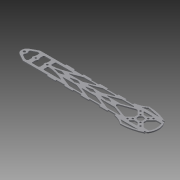
# Autodesk Inventor part: Arm
Saved by Autodesk Inventor 2014 SP1 (Build 180222100, 222)
## iProperties
Created: 2014-07-26
Part Number: Arm
Material: Generic
Document SubType Name: Modeling
Designer: Ryan
Density: 1 g/cm^3
Appearance: Default
Author: Ryan
Autodesk Inventor part; units mm, degrees
ref_plane "YZ Plane" through (0, 0, 0) normal (1, 0, 0) x (0, 1, 0)
ref_plane "XZ Plane" through (0, 0, 0) normal (0, 1, 0) x (-1, 0, 0)
ref_plane "XY Plane" through (0, 0, 0) normal (0, 0, 1) x (1, 0, 0)
sketch "DWG" plane through (0, 0, 0) normal (0, 0, 1) x (1, 0, 0)
  arc A0 (4.5611, 40.079) -> (0, 25.5088) centre (25.5524, 25.5088) ccw construction
  arc A1 (5.3826, 40.5088) -> (4.5611, 40.079) centre (5.3826, 39.5088) ccw construction
  line L0 (5.3826, 40.5088) -> (8.9844, 40.5088) construction
  line L1 (8.9844, 42.5088) -> (5.9833, 42.5088) construction
  arc A2 (41.2735, 51.0175) -> (5.9833, 42.5088) centre (43.8792, -37.2276) ccw construction
  arc A3 (41.2735, 51.0175) -> (59.244, 43.0088) centre (65.3633, 80.9055) ccw construction
  line L2 (222.3706, 39.9043) -> (233.741, 33.7395) construction
  line L3 (177.3927, 40.5088) -> (219.9874, 40.5088) construction
  arc A4 (222.3706, 39.9043) -> (219.9874, 40.5088) centre (219.9874, 35.5088) ccw construction
  arc A5 (0, 25.5088) -> (4.5611, 10.9385) centre (25.5524, 25.5088) ccw construction
  arc A6 (4.5611, 10.9385) -> (5.3826, 10.5088) centre (5.3826, 11.5088) ccw construction
  line L4 (5.3826, 10.5088) -> (8.9839, 10.5088) construction
  line L5 (8.9838, 8.5088) -> (5.9875, 8.5088) construction
  arc A7 (5.9875, 8.5088) -> (41.2735, 0) centre (43.8737, 88.2038) ccw construction
  arc A8 (59.244, 8.0088) -> (41.2735, 0) centre (65.3633, -29.888) ccw construction
  line L6 (222.3706, 11.1132) -> (233.741, 17.278) construction
  line L7 (177.3921, 10.5093) -> (219.9874, 10.5088) construction
  arc A9 (219.9874, 10.5088) -> (222.3706, 11.1132) centre (219.9874, 15.5088) ccw construction
  circle A10 centre (37.7725, 32.248) radius 1.6 construction
  circle A11 centre (24.3375, 18.813) radius 1.6 construction
  circle A12 centre (25.3982, 31.1874) radius 1.6 construction
  circle A13 centre (36.7119, 19.8736) radius 1.6 construction
  circle A14 centre (31.055, 25.5117) radius 5 construction
  line L8 (6.7874, 36.5088) -> (12.7618, 36.5088) construction
  arc A15 (16.2903, 35.0513) -> (12.7618, 36.5088) centre (12.7618, 31.5088) ccw construction
  line L9 (6.7874, 14.5088) -> (12.7425, 14.5088) construction
  arc A16 (12.7425, 14.5088) -> (16.278, 15.9732) centre (12.7425, 19.5088) ccw construction
  circle A17 centre (233.741, 25.5088) radius 2.1 construction
  circle A18 centre (193.7046, 25.5088) radius 1.6 construction
  circle A19 centre (213.981, 25.5088) radius 1.6 construction
  line L10 (199.0246, 36.3758) -> (208.661, 36.3758) construction
  arc A20 (199.0246, 36.3758) -> (197.1246, 34.4758) centre (199.0246, 34.4758) ccw construction
  line L11 (197.1246, 34.4758) -> (197.1246, 28.9288) construction
  line L12 (210.561, 28.9288) -> (210.561, 34.4758) construction
  arc A21 (210.561, 34.4758) -> (208.661, 36.3758) centre (208.661, 34.4758) ccw construction
  line L13 (199.0246, 14.6417) -> (208.661, 14.6417) construction
  arc A22 (197.1246, 16.5417) -> (199.0246, 14.6417) centre (199.0246, 16.5417) ccw construction
  line L14 (197.1246, 16.5417) -> (197.1246, 22.0888) construction
  line L15 (210.561, 22.0888) -> (210.561, 16.5417) construction
  arc A23 (208.661, 14.6417) -> (210.561, 16.5417) centre (208.661, 16.5417) ccw construction
  arc A24 (197.1246, 22.0888) -> (197.1246, 28.9288) centre (193.6586, 25.5088) ccw construction
  arc A25 (210.561, 28.9288) -> (210.561, 22.0888) centre (213.981, 25.5088) ccw construction
  line L16 (221.1675, 36.3758) -> (219.301, 36.3758) construction
  line L17 (217.401, 28.9288) -> (217.401, 34.4758) construction
  arc A26 (219.301, 36.3758) -> (217.401, 34.4758) centre (219.301, 34.4758) ccw construction
  arc A27 (217.401, 22.0888) -> (217.401, 28.9288) centre (213.981, 25.5088) ccw construction
  line L18 (222.0731, 36.1461) -> (229.3266, 32.2135) construction
  arc A28 (222.0731, 36.1461) -> (221.1675, 36.3758) centre (221.1675, 34.4758) ccw construction
  line L19 (230.321, 30.5432) -> (230.321, 28.9288) construction
  arc A29 (230.321, 30.5432) -> (229.3266, 32.2135) centre (228.421, 30.5432) ccw construction
  arc A30 (230.321, 28.9288) -> (230.321, 22.0888) centre (233.741, 25.5088) ccw construction
  line L20 (221.1675, 14.6417) -> (219.301, 14.6417) construction
  line L21 (217.401, 22.0888) -> (217.401, 16.5417) construction
  arc A31 (217.401, 16.5417) -> (219.301, 14.6417) centre (219.301, 16.5417) ccw construction
  line L22 (222.0731, 14.8714) -> (229.3266, 18.804) construction
  arc A32 (221.1675, 14.6417) -> (222.0731, 14.8714) centre (221.1675, 16.5417) ccw construction
  line L23 (230.321, 20.4743) -> (230.321, 22.0888) construction
  arc A33 (229.3266, 18.804) -> (230.321, 20.4743) centre (228.421, 20.4743) ccw construction
  arc A34 (233.741, 17.278) -> (233.741, 33.7395) centre (229.1559, 25.5088) ccw construction
  line L24 (16.9699, 44.0088) -> (46.9493, 44.0088) construction
  arc A35 (40.3396, 48.7188) -> (16.9395, 44.204) centre (47.756, -52.6194) ccw construction
  arc A36 (16.9395, 44.204) -> (16.9699, 44.0088) centre (16.9699, 44.1088) ccw construction
  arc A37 (40.4838, 48.6716) -> (46.9971, 44.1966) centre (65.3633, 77.9055) ccw construction
  arc A38 (40.4838, 48.6716) -> (40.3396, 48.7188) centre (40.3542, 48.5193) ccw construction
  arc A39 (46.9493, 44.0088) -> (46.9971, 44.1966) centre (46.9493, 44.1088) ccw construction
  line L25 (16.9699, 7.0088) -> (46.9493, 7.0088) construction
  arc A40 (16.9395, 6.8135) -> (40.3396, 2.2987) centre (47.756, 103.637) ccw construction
  arc A41 (16.9699, 7.0088) -> (16.9395, 6.8135) centre (16.9699, 6.9088) ccw construction
  arc A42 (40.3396, 2.2987) -> (40.4838, 2.3459) centre (40.3542, 2.4982) ccw construction
  arc A43 (46.9971, 6.8209) -> (40.4838, 2.3459) centre (65.3633, -26.888) ccw construction
  arc A44 (46.9971, 6.8209) -> (46.9493, 7.0088) centre (46.9493, 6.9088) ccw construction
  circle A45 centre (19.7413, 36.8442) radius 1.6 construction
  circle A46 centre (42.3687, 36.8442) radius 1.6 construction
  circle A47 centre (19.7413, 14.2168) radius 1.6 construction
  circle A48 centre (42.3687, 14.2168) radius 1.6 construction
  arc A49 (88.4057, 36.5567) -> (104.0793, 30.6226) centre (168.1638, 223.554) ccw construction
  arc A50 (104.0793, 30.6226) -> (104.7095, 30.5207) centre (104.7098, 32.5207) ccw construction
  arc A51 (88.7983, 38.4766) -> (88.4057, 36.5567) centre (88.798, 37.4766) ccw construction
  arc A52 (109.7552, 38.3866) -> (127.7097, 31.4923) centre (191.5259, 224.5125) ccw construction
  arc A53 (127.5526, 30.5176) -> (127.7097, 31.4923) centre (127.5527, 31.0176) ccw construction
  arc A54 (109.7552, 38.3866) -> (109.3532, 38.4711) centre (109.353, 37.4711) ccw construction
  line L26 (88.7983, 38.4766) -> (109.3532, 38.4711) construction
  arc A55 (55.2642, 36.5656) -> (71.1057, 30.5758) centre (135.0223, 223.5628) ccw construction
  arc A56 (71.1057, 30.5758) -> (71.42, 30.5251) centre (71.4201, 31.5251) ccw construction
  arc A57 (55.6568, 38.4854) -> (55.2642, 36.5656) centre (55.6565, 37.4854) ccw construction
  arc A58 (76.6137, 38.3955) -> (94.5815, 31.4968) centre (158.3844, 224.5214) ccw construction
  arc A59 (94.4246, 30.522) -> (94.5815, 31.4968) centre (94.4246, 31.022) ccw construction
  arc A60 (76.6137, 38.3955) -> (76.2117, 38.4799) centre (76.2115, 37.4799) ccw construction
  line L27 (55.6568, 38.4854) -> (76.2117, 38.4799) construction
  arc A61 (121.5472, 36.5479) -> (137.2074, 30.6182) centre (201.3053, 223.5451) ccw construction
  arc A62 (137.2074, 30.6182) -> (137.8377, 30.5162) centre (137.838, 32.5162) ccw construction
  arc A63 (121.9398, 38.4677) -> (121.5472, 36.5479) centre (121.9395, 37.4677) ccw construction
  arc A64 (142.8967, 38.3777) -> (160.8378, 31.4879) centre (224.6674, 224.5037) ccw construction
  arc A65 (160.6807, 30.5132) -> (160.8378, 31.4879) centre (160.6808, 31.0132) ccw construction
  arc A66 (142.8967, 38.3777) -> (142.4947, 38.4622) centre (142.4945, 37.4622) ccw construction
  line L28 (121.9398, 38.4677) -> (142.4947, 38.4622) construction
  arc A67 (160.1468, 15.6085) -> (160.3303, 14.6434) centre (160.3303, 15.1434) ccw construction
  line L29 (160.3303, 14.6434) -> (188.3846, 14.6417) construction
  arc A68 (160.3303, 36.3741) -> (160.1468, 35.409) centre (160.3303, 35.8741) ccw construction
  arc A69 (160.1468, 35.409) -> (188.105, 27.8173) centre (195.5628, 110.559) ccw construction
  arc A70 (188.105, 27.8173) -> (190.2846, 29.8092) centre (188.2846, 29.8092) ccw construction
  line L30 (160.3303, 36.3741) -> (188.3846, 36.3758) construction
  arc A71 (170.2297, 28.0978) -> (164.315, 25.9784) centre (235.8427, -164.3191) ccw construction
  arc A72 (164.3149, 25.0423) -> (170.2313, 22.9205) centre (235.8946, 215.3202) ccw construction
  arc A73 (170.2313, 22.9205) -> (171.4285, 22.8907) centre (170.8773, 24.8133) ccw construction
  arc A74 (164.315, 25.9784) -> (164.3149, 25.0423) centre (164.491, 25.5103) ccw construction
  arc A75 (4.9392, 35.273) -> (3, 25.5088) centre (28.5524, 25.5088) ccw construction
  arc A76 (6.7874, 36.5088) -> (4.9392, 35.273) centre (6.7874, 34.5088) ccw construction
  arc A77 (3, 25.5088) -> (4.9392, 15.7445) centre (28.5524, 25.5088) ccw construction
  arc A78 (4.9392, 15.7445) -> (6.7874, 14.5088) centre (6.7874, 16.5088) ccw construction
  line L31 (24.7107, 39.5088) -> (37.3994, 39.5088) construction
  arc A79 (24.7107, 39.5088) -> (24.0036, 37.8016) centre (24.7107, 38.5088) ccw construction
  arc A80 (38.1065, 37.8016) -> (37.3994, 39.5088) centre (37.3994, 38.5088) ccw construction
  arc A81 (32.6348, 33.5927) -> (29.4753, 33.5927) centre (31.055, 25.7502) ccw construction
  arc A82 (27.6661, 34.1391) -> (29.4753, 33.5927) centre (29.0804, 35.5533) ccw construction
  arc A83 (32.6348, 33.5927) -> (34.4439, 34.1391) centre (33.0297, 35.5533) ccw construction
  line L32 (24.0036, 37.8016) -> (27.6661, 34.1391) construction
  line L33 (38.1065, 37.8016) -> (34.4439, 34.1391) construction
  line L34 (24.7107, 11.5523) -> (37.3994, 11.5523) construction
  arc A84 (24.0036, 13.2594) -> (24.7107, 11.5523) centre (24.7107, 12.5523) ccw construction
  arc A85 (37.3994, 11.5523) -> (38.1065, 13.2594) centre (37.3994, 12.5523) ccw construction
  arc A86 (29.4753, 17.4683) -> (32.6348, 17.4683) centre (31.055, 25.3108) ccw construction
  arc A87 (29.4753, 17.4683) -> (27.6661, 16.9219) centre (29.0804, 15.5077) ccw construction
  arc A88 (34.4439, 16.9219) -> (32.6348, 17.4683) centre (33.0297, 15.5077) ccw construction
  line L35 (24.0036, 13.2594) -> (27.6661, 16.9219) construction
  line L36 (38.1065, 13.2594) -> (34.4439, 16.9219) construction
  line L37 (39.6636, 28.9194) -> (45.5743, 34.8301) construction
  line L38 (39.6636, 22.1416) -> (45.5743, 16.2309) construction
  line L39 (16.2903, 35.0513) -> (22.4464, 28.9194) construction
  arc A89 (39.1172, 23.9508) -> (39.1172, 27.1102) centre (31.2747, 25.5305) ccw construction
  arc A90 (39.1172, 23.9508) -> (39.6636, 22.1416) centre (41.0778, 23.5558) ccw construction
  arc A91 (39.6636, 28.9194) -> (39.1172, 27.1102) centre (41.0778, 27.5052) ccw construction
  arc A92 (22.9928, 27.1102) -> (22.9928, 23.9508) centre (30.8353, 25.5305) ccw construction
  arc A93 (22.4464, 22.1416) -> (22.9928, 23.9508) centre (21.0322, 23.5558) ccw construction
  arc A94 (22.9928, 27.1102) -> (22.4464, 28.9194) centre (21.0322, 27.5052) ccw construction
  line L40 (16.278, 15.9732) -> (22.4464, 22.1416) construction
  arc A95 (49.8854, 35.7167) -> (45.5743, 34.8301) centre (48.4027, 32.0016) ccw construction
  arc A96 (45.5743, 16.2309) -> (49.8854, 15.3443) centre (48.4027, 19.0594) ccw construction
  arc A97 (104.078, 20.4189) -> (88.4027, 14.4889) centre (168.1108, -172.5296) ccw construction
  arc A98 (104.7082, 20.5207) -> (104.078, 20.4189) centre (104.7079, 18.5207) ccw construction
  arc A99 (88.4027, 14.4889) -> (88.7948, 12.569) centre (88.7948, 13.569) ccw construction
  arc A100 (127.7081, 19.5428) -> (109.7517, 12.6534) centre (191.4727, -173.4945) ccw construction
  arc A101 (127.7081, 19.5428) -> (127.5513, 20.5176) centre (127.5512, 20.0176) ccw construction
  arc A102 (109.3498, 12.569) -> (109.7517, 12.6534) centre (109.3498, 13.569) ccw construction
  line L41 (88.7948, 12.569) -> (109.3498, 12.569) construction
  arc A103 (70.95, 20.4233) -> (55.2612, 14.4889) centre (134.9693, -172.5296) ccw construction
  arc A104 (71.58, 20.5251) -> (70.95, 20.4233) centre (71.5798, 18.5251) ccw construction
  arc A105 (55.2612, 14.4889) -> (55.6533, 12.569) centre (55.6533, 13.569) ccw construction
  arc A106 (94.5799, 19.5472) -> (76.6102, 12.6534) centre (158.3312, -173.4945) ccw construction
  arc A107 (94.5799, 19.5472) -> (94.4232, 20.522) centre (94.4231, 20.022) ccw construction
  arc A108 (76.2083, 12.569) -> (76.6102, 12.6534) centre (76.2083, 13.569) ccw construction
  line L42 (55.6533, 12.569) -> (76.2083, 12.569) construction
  arc A109 (137.206, 20.4144) -> (121.5442, 14.4889) centre (201.2523, -172.5296) ccw construction
  arc A110 (137.8364, 20.5162) -> (137.206, 20.4144) centre (137.8361, 18.5162) ccw construction
  arc A111 (121.5442, 14.4889) -> (121.9363, 12.569) centre (121.9363, 13.569) ccw construction
  arc A112 (160.8362, 19.5384) -> (142.8932, 12.6534) centre (224.6142, -173.4945) ccw construction
  arc A113 (160.8362, 19.5384) -> (160.6794, 20.5132) centre (160.6793, 20.0132) ccw construction
  arc A114 (142.4913, 12.569) -> (142.8932, 12.6534) centre (142.4913, 13.569) ccw construction
  line L43 (121.9363, 12.569) -> (142.4913, 12.569) construction
  line L44 (71.42, 30.5251) -> (94.4246, 30.522) construction
  line L45 (104.7095, 30.5207) -> (127.5526, 30.5176) construction
  line L46 (137.8377, 30.5162) -> (160.6807, 30.5132) construction
  line L47 (71.58, 20.5251) -> (94.4232, 20.522) construction
  line L48 (104.7082, 20.5207) -> (127.5513, 20.5176) construction
  line L49 (137.8364, 20.5162) -> (160.6794, 20.5132) construction
  arc A115 (190.2846, 34.4758) -> (188.3846, 36.3758) centre (188.3846, 34.4758) ccw construction
  line L50 (190.2846, 34.4758) -> (190.2846, 29.8092) construction
  arc A116 (188.3846, 14.6417) -> (190.2846, 16.5417) centre (188.3846, 16.5417) ccw construction
  line L51 (190.2846, 16.5417) -> (190.2846, 21.2083) construction
  arc A117 (171.4264, 28.1274) -> (180.7426, 26.0016) centre (195.4354, 111.8692) ccw construction
  arc A118 (171.4264, 28.1274) -> (170.2297, 28.0978) centre (170.8752, 26.2048) ccw construction
  arc A119 (180.7426, 25.0159) -> (171.4285, 22.8907) centre (195.4354, -60.8517) ccw construction
  arc A120 (180.7426, 25.0159) -> (180.7426, 26.0016) centre (180.6583, 25.5088) ccw construction
  arc A121 (188.105, 23.2002) -> (160.1468, 15.6085) centre (195.5628, -59.5415) ccw construction
  arc A122 (190.2846, 21.2083) -> (188.105, 23.2002) centre (188.2846, 21.2083) ccw construction
  arc A123 (143.0624, 28.1018) -> (137.1477, 25.9823) centre (208.6754, -164.3151) ccw construction
  arc A124 (137.1476, 25.0463) -> (143.064, 22.9245) centre (208.7272, 215.3242) ccw construction
  arc A125 (143.064, 22.9245) -> (144.2612, 22.8947) centre (143.71, 24.8173) ccw construction
  arc A126 (137.1477, 25.9823) -> (137.1476, 25.0463) centre (137.3236, 25.5143) ccw construction
  arc A127 (144.2591, 28.1314) -> (153.5753, 26.0056) centre (168.2681, 111.8732) ccw construction
  arc A128 (144.2591, 28.1314) -> (143.0624, 28.1018) centre (143.7079, 26.2088) ccw construction
  arc A129 (153.5753, 25.0199) -> (144.2612, 22.8947) centre (168.2681, -60.8477) ccw construction
  arc A130 (153.5753, 25.0199) -> (153.5753, 26.0056) centre (153.491, 25.5127) ccw construction
  arc A131 (115.8951, 28.1058) -> (109.9804, 25.9863) centre (181.5081, -164.3111) ccw construction
  arc A132 (109.9803, 25.0503) -> (115.8967, 22.9284) centre (181.5599, 215.3282) ccw construction
  arc A133 (115.8967, 22.9284) -> (117.0938, 22.8987) centre (116.5427, 24.8212) ccw construction
  arc A134 (109.9804, 25.9863) -> (109.9803, 25.0503) centre (110.1563, 25.5183) ccw construction
  arc A135 (117.0917, 28.1353) -> (126.408, 26.0095) centre (141.1008, 111.8772) ccw construction
  arc A136 (117.0917, 28.1353) -> (115.8951, 28.1058) centre (116.5406, 26.2128) ccw construction
  arc A137 (126.408, 25.0239) -> (117.0938, 22.8987) centre (141.1007, -60.8437) ccw construction
  arc A138 (126.408, 25.0239) -> (126.408, 26.0095) centre (126.3236, 25.5167) ccw construction
  arc A139 (88.7277, 28.1097) -> (82.8131, 25.9903) centre (154.3407, -164.3072) ccw construction
  arc A140 (82.8129, 25.0543) -> (88.7294, 22.9324) centre (154.3926, 215.3321) ccw construction
  arc A141 (88.7294, 22.9324) -> (89.9265, 22.9026) centre (89.3754, 24.8252) ccw construction
  arc A142 (82.8131, 25.9903) -> (82.8129, 25.0543) centre (82.989, 25.5222) ccw construction
  arc A143 (89.9244, 28.1393) -> (99.2406, 26.0135) centre (113.9334, 111.8812) ccw construction
  arc A144 (89.9244, 28.1393) -> (88.7277, 28.1097) centre (89.3732, 26.2168) ccw construction
  arc A145 (99.2406, 25.0278) -> (89.9265, 22.9026) centre (113.9334, -60.8398) ccw construction
  arc A146 (99.2406, 25.0278) -> (99.2406, 26.0135) centre (99.1563, 25.5207) ccw construction
  arc A147 (71.4561, 23.1317) -> (49.8854, 15.3443) centre (129.5935, -171.6742) ccw construction
  arc A148 (49.8854, 35.7167) -> (71.4567, 27.9227) centre (129.6435, 222.7139) ccw construction
  arc A149 (71.4561, 23.1317) -> (71.4567, 27.9227) centre (70.7412, 25.5273) ccw construction
  line L52 (59.244, 43.0088) -> (59.244, 40.5088) construction
  line L53 (59.244, 40.5088) -> (72.2147, 40.5088) construction
  line L54 (72.2147, 40.5088) -> (72.2147, 42.5088) construction
  line L55 (72.2147, 42.5088) -> (86.3318, 42.5088) construction
  line L56 (86.3318, 42.5088) -> (86.3318, 40.5088) construction
  line L57 (86.3318, 40.5088) -> (104.7173, 40.5088) construction
  line L58 (119.0249, 40.5088) -> (132.7899, 40.5088) construction
  line L59 (147.3354, 40.5088) -> (162.685, 40.5088) construction
  line L60 (104.7173, 40.5088) -> (104.7173, 42.5088) construction
  line L61 (104.7173, 42.5088) -> (119.0249, 42.5088) construction
  line L62 (119.0249, 42.5088) -> (119.0249, 40.5088) construction
  line L63 (132.7899, 40.5088) -> (132.7899, 42.5088) construction
  line L64 (132.7899, 42.5088) -> (147.3354, 42.5088) construction
  line L65 (147.3354, 42.5088) -> (147.3354, 40.5088) construction
  line L66 (162.685, 40.5088) -> (162.685, 42.5088) construction
  line L67 (162.685, 42.5088) -> (177.3927, 42.5088) construction
  line L68 (177.3927, 42.5088) -> (177.3927, 40.5088) construction
  line L69 (8.9844, 40.5088) -> (8.9844, 42.5088) construction
  line L70 (59.244, 8.0088) -> (59.2434, 10.5136) construction
  line L71 (59.2434, 10.5136) -> (72.2142, 10.5131) construction
  line L72 (72.2142, 10.5131) -> (72.2141, 8.5131) construction
  line L73 (72.2141, 8.5131) -> (86.3312, 8.5126) construction
  line L74 (86.3312, 8.5126) -> (86.3312, 10.5126) construction
  line L75 (86.3312, 10.5126) -> (104.7167, 10.512) construction
  line L76 (119.0244, 10.5114) -> (132.7893, 10.5109) construction
  line L77 (147.3349, 10.5104) -> (162.6844, 10.5099) construction
  line L78 (104.7167, 10.512) -> (104.7166, 8.512) construction
  line L79 (104.7166, 8.512) -> (119.0243, 8.5114) construction
  line L80 (119.0243, 8.5114) -> (119.0244, 10.5114) construction
  line L81 (132.7893, 10.511) -> (132.7892, 8.511) construction
  line L82 (132.7892, 8.511) -> (147.3348, 8.5104) construction
  line L83 (147.3348, 8.5104) -> (147.3349, 10.5104) construction
  line L84 (162.6844, 10.5099) -> (162.6844, 8.5099) construction
  line L85 (162.6844, 8.5099) -> (177.3921, 8.5093) construction
  line L86 (177.3921, 8.5093) -> (177.3921, 10.5093) construction
  line L87 (8.9839, 10.5088) -> (8.9838, 8.5088) construction
  point P0 (110.4936, 25.5142)
sketch "Sketch1" plane through (0, 0, 0) normal (0, 1, 0) x (-1, 0, 0)
  circle A0 centre (31.055, 25.5117) radius 5
  line L0 (72.2147, 42.5088) -> (86.3318, 42.5088)
  line L1 (72.2147, 42.5088) -> (72.2147, 40.5088)
  line L2 (72.2147, 40.5088) -> (59.244, 40.5088)
  line L3 (59.244, 40.5088) -> (59.244, 43.0088)
  line L4 (86.3318, 42.5088) -> (86.3318, 40.5088)
  line L5 (86.3318, 40.5088) -> (104.7173, 40.5038)
  line L6 (104.7173, 40.5038) -> (104.7173, 42.5088)
  line L7 (104.7173, 42.5088) -> (119.0249, 42.5088)
  line L8 (119.0249, 42.5088) -> (119.0249, 40.5088)
  line L9 (119.0249, 40.5088) -> (132.7899, 40.5088)
  line L10 (132.7899, 40.5088) -> (132.7899, 42.5088)
  line L11 (132.7899, 42.5088) -> (147.3354, 42.5088)
  line L12 (147.3354, 42.5088) -> (147.3354, 40.5088)
  line L13 (147.3354, 40.5088) -> (162.685, 40.5088)
  line L14 (162.685, 40.5088) -> (162.685, 42.5088)
  line L15 (162.685, 42.5088) -> (177.3927, 42.5088)
  line L16 (177.3927, 42.5088) -> (177.3927, 40.5088)
  line L17 (59.244, 8.0088) -> (59.244, 10.5136)
  line L18 (59.244, 10.5136) -> (72.2142, 10.5136)
  line L19 (72.2142, 10.5136) -> (72.2142, 8.5131)
  line L20 (72.2142, 8.5131) -> (86.3312, 8.5131)
  line L21 (86.3312, 8.5131) -> (86.3312, 10.5195)
  line L22 (86.3312, 10.5195) -> (104.7167, 10.5234)
  line L23 (104.7167, 10.5234) -> (104.7171, 8.512)
  line L24 (104.7171, 8.512) -> (119.0243, 8.5151)
  line L25 (119.0243, 8.5151) -> (119.0239, 10.5114)
  line L26 (119.0239, 10.5114) -> (132.7893, 10.5295)
  line L27 (132.7893, 10.5295) -> (132.7919, 8.511)
  line L28 (132.7919, 8.511) -> (147.3348, 8.5104)
  line L29 (147.3348, 8.5104) -> (147.3349, 10.5104)
  line L30 (147.3349, 10.5104) -> (162.6844, 10.5359)
  line L31 (162.6844, 10.5359) -> (162.6878, 8.5099)
  line L32 (162.6878, 8.5099) -> (177.3921, 8.5093)
  line L33 (177.3921, 8.5093) -> (177.3921, 10.5093)
  line L34 (71.42, 30.5251) -> (94.4246, 30.522)
  line L35 (55.6568, 38.4854) -> (76.2117, 38.4799)
  arc A1 (94.4246, 30.522) -> (94.5815, 31.4968) centre (94.4246, 31.022) ccw
  arc A2 (76.6137, 38.3955) -> (76.2117, 38.4799) centre (76.2115, 37.4799) ccw
  line L36 (76.6137, 38.3955) -> (94.5815, 31.4968)
  arc A3 (55.6568, 38.4854) -> (55.2642, 36.5656) centre (55.6565, 37.4854) ccw
  arc A4 (71.1057, 30.5758) -> (71.42, 30.5251) centre (71.4201, 31.5251) ccw
  line L37 (71.1057, 30.5758) -> (55.2642, 36.5656)
  line L38 (217.401, 28.9288) -> (217.401, 34.4758)
  circle A5 centre (193.7046, 25.5088) radius 1.6
  circle A6 centre (213.981, 25.5088) radius 1.6
  circle A7 centre (233.741, 25.5088) radius 2.1
  line L39 (210.561, 28.9288) -> (210.561, 34.4758)
  line L40 (210.561, 22.0888) -> (210.561, 16.5417)
  line L41 (217.401, 22.0888) -> (217.401, 16.5417)
  line L42 (221.249, 14.6434) -> (219.2195, 14.6434)
  line L43 (208.661, 14.6417) -> (199.0246, 14.6417)
  line L44 (197.1246, 16.5417) -> (197.1246, 22.0888)
  line L45 (197.1246, 28.9288) -> (197.1246, 34.4758)
  line L46 (199.0246, 36.3758) -> (208.661, 36.3758)
  line L47 (219.301, 36.3758) -> (221.1675, 36.3758)
  line L48 (230.321, 28.9288) -> (230.321, 30.5432)
  line L49 (230.321, 22.0888) -> (230.321, 20.4743)
  arc A8 (197.1246, 22.0888) -> (197.1246, 28.9288) centre (193.6586, 25.5088) ccw
  arc A9 (210.561, 28.9288) -> (210.561, 22.0888) centre (213.981, 25.5088) ccw
  arc A10 (217.401, 22.0888) -> (217.401, 28.9288) centre (213.981, 25.5088) ccw
  arc A11 (210.561, 34.4758) -> (208.661, 36.3758) centre (208.661, 34.4758) ccw
  arc A12 (199.0246, 36.3758) -> (197.1246, 34.4758) centre (199.0246, 34.4758) ccw
  arc A13 (197.1246, 16.5417) -> (199.0246, 14.6417) centre (199.0246, 16.5417) ccw
  arc A14 (208.661, 14.6417) -> (210.561, 16.5417) centre (208.661, 16.5417) ccw
  arc A15 (217.401, 16.5417) -> (219.2195, 14.6434) centre (219.301, 16.5417) ccw
  arc A16 (221.249, 14.6434) -> (222.0731, 14.8714) centre (221.1675, 16.5417) ccw
  arc A17 (230.321, 28.9288) -> (230.321, 22.0888) centre (233.741, 25.5088) ccw
  arc A18 (230.321, 30.5432) -> (229.3266, 32.2135) centre (228.421, 30.5432) ccw
  arc A19 (219.301, 36.3758) -> (217.401, 34.4758) centre (219.301, 34.4758) ccw
  arc A20 (222.0731, 36.1461) -> (221.1675, 36.3758) centre (221.1675, 34.4758) ccw
  line L50 (222.0731, 36.1461) -> (229.3266, 32.2135)
  arc A21 (229.3266, 18.804) -> (230.321, 20.4743) centre (228.421, 20.4743) ccw
  line L51 (222.0731, 14.8714) -> (229.3266, 18.804)
  arc A22 (219.9874, 10.5088) -> (222.3706, 11.1132) centre (219.9874, 15.5088) ccw
  arc A23 (233.741, 17.278) -> (233.741, 33.7395) centre (229.1559, 25.5088) ccw
  arc A24 (222.3706, 39.9043) -> (219.9874, 40.5088) centre (219.9874, 35.5088) ccw
  line L52 (222.3706, 39.9043) -> (233.741, 33.7395)
  line L53 (222.3706, 11.1132) -> (233.741, 17.278)
  line L54 (219.9874, 10.5088) -> (177.3921, 10.5093)
  line L55 (177.3927, 40.5088) -> (219.9874, 40.5088)
  circle A25 centre (24.3375, 18.813) radius 1.6
  circle A26 centre (36.7119, 19.8736) radius 1.6
  circle A27 centre (42.3687, 14.2168) radius 1.6
  circle A28 centre (19.7413, 14.2168) radius 1.6
  circle A29 centre (25.3982, 31.1874) radius 1.6
  circle A30 centre (37.7725, 32.248) radius 1.6
  circle A31 centre (42.3687, 36.8442) radius 1.6
  circle A32 centre (19.7413, 36.8442) radius 1.6
  arc A33 (5.3826, 40.5088) -> (4.5611, 40.079) centre (5.3826, 39.5088) ccw
  line L56 (5.3826, 40.5088) -> (8.9844, 40.5088)
  line L57 (8.9844, 40.5088) -> (8.9844, 42.5088)
  line L58 (5.9833, 42.5088) -> (8.9844, 42.5088)
  line L59 (8.9839, 10.5088) -> (8.9838, 8.5088)
  line L60 (5.9875, 8.5088) -> (8.9838, 8.5088)
  arc A34 (4.5611, 10.9385) -> (5.3826, 10.5088) centre (5.3826, 11.5088) ccw
  line L61 (5.3826, 10.5088) -> (8.9839, 10.5088)
  arc A35 (4.5611, 40.079) -> (4.5611, 10.9385) centre (25.5524, 25.5088) ccw
  arc A36 (41.2735, 51.0175) -> (59.244, 43.0088) centre (65.3633, 80.9055) ccw
  arc A37 (59.244, 8.0088) -> (41.2735, 0) centre (65.3633, -29.888) ccw
  arc A38 (22.9928, 27.1102) -> (22.4464, 28.9194) centre (21.0322, 27.5052) ccw
  arc A39 (22.4464, 22.1416) -> (22.9928, 23.9508) centre (21.0322, 23.5558) ccw
  arc A40 (12.7425, 14.5088) -> (16.278, 15.9732) centre (12.7425, 19.5088) ccw
  arc A41 (16.2903, 35.0513) -> (12.7618, 36.5088) centre (12.7618, 31.5088) ccw
  arc A42 (6.7874, 36.5088) -> (4.9392, 35.273) centre (6.7874, 34.5088) ccw
  arc A43 (4.9392, 15.7445) -> (6.7874, 14.5088) centre (6.7874, 16.5088) ccw
  arc A44 (4.9392, 35.273) -> (4.9392, 15.7445) centre (28.5524, 25.5088) ccw
  line L62 (12.7425, 14.5088) -> (6.7874, 14.5088)
  line L63 (16.278, 15.9732) -> (22.4464, 22.1416)
  line L64 (22.4464, 28.9194) -> (16.2903, 35.0513)
  line L65 (12.7618, 36.5088) -> (6.7874, 36.5088)
  arc A45 (16.9395, 44.204) -> (16.9699, 44.0088) centre (16.9699, 44.1088) ccw
  arc A46 (40.4838, 48.6716) -> (40.3542, 48.7193) centre (40.3542, 48.5193) ccw
  arc A47 (46.9493, 44.0088) -> (46.9971, 44.1966) centre (46.9493, 44.1088) ccw
  line L66 (46.9971, 44.1966) -> (40.4838, 48.6716)
  arc A48 (40.3542, 48.7193) -> (16.9395, 44.204) centre (47.7453, -52.5759) ccw
  line L67 (46.9493, 44.0088) -> (16.9699, 44.0088)
  arc A49 (71.4561, 23.1317) -> (71.4567, 27.9227) centre (70.7412, 25.5273) ccw
  arc A50 (39.6636, 28.9194) -> (39.1172, 27.1102) centre (41.0778, 27.5052) ccw
  arc A51 (39.1172, 23.9508) -> (39.6636, 22.1416) centre (41.0778, 23.5558) ccw
  arc A52 (49.8854, 35.7167) -> (45.5743, 34.8301) centre (48.4027, 32.0016) ccw
  arc A53 (45.5743, 16.2309) -> (49.8854, 15.3443) centre (48.4027, 19.0594) ccw
  line L68 (39.6636, 28.9194) -> (45.5743, 34.8301)
  line L69 (71.4567, 27.9227) -> (49.8854, 35.7167)
  line L70 (71.4561, 23.1317) -> (49.8854, 15.3443)
  line L71 (39.6636, 22.1416) -> (45.5743, 16.2309)
  arc A54 (39.1172, 23.9508) -> (39.1172, 27.1102) centre (31.2747, 25.5305) ccw
  arc A55 (34.4439, 16.9219) -> (32.6348, 17.4683) centre (33.0297, 15.5077) ccw
  arc A56 (29.4753, 17.4683) -> (27.6661, 16.9219) centre (29.0804, 15.5077) ccw
  arc A57 (29.4753, 17.4683) -> (32.6348, 17.4683) centre (31.055, 25.3108) ccw
  arc A58 (24.0036, 13.2594) -> (24.7107, 11.5523) centre (24.7107, 12.5523) ccw
  arc A59 (37.3994, 11.5523) -> (38.1065, 13.2594) centre (37.3994, 12.5523) ccw
  line L72 (24.7107, 11.5523) -> (37.3994, 11.5523)
  line L73 (38.1065, 13.2594) -> (34.4439, 16.9219)
  line L74 (27.6661, 16.9219) -> (24.0036, 13.2594)
  arc A60 (27.6661, 34.1391) -> (29.4753, 33.5927) centre (29.0804, 35.5533) ccw
  arc A61 (32.6348, 33.5927) -> (34.4439, 34.1391) centre (33.0297, 35.5533) ccw
  arc A62 (32.6348, 33.5927) -> (29.4753, 33.5927) centre (31.055, 25.7502) ccw
  arc A63 (38.1065, 37.8016) -> (37.3994, 39.5088) centre (37.3994, 38.5088) ccw
  arc A64 (24.7107, 39.5088) -> (24.0036, 37.8016) centre (24.7107, 38.5088) ccw
  line L75 (38.1065, 37.8016) -> (34.4439, 34.1391)
  line L76 (27.6661, 34.1391) -> (24.0036, 37.8016)
  line L77 (24.7107, 39.5088) -> (37.3994, 39.5088)
  arc A65 (46.9971, 6.8209) -> (46.9493, 7.0088) centre (46.9493, 6.9088) ccw
  arc A66 (40.3396, 2.2987) -> (40.4838, 2.3459) centre (40.3542, 2.4982) ccw
  arc A67 (16.9699, 7.0088) -> (16.9395, 6.8135) centre (16.9699, 6.9088) ccw
  line L78 (16.9699, 7.0088) -> (46.9493, 7.0088)
  line L79 (40.4838, 2.3459) -> (46.9971, 6.8209)
  arc A68 (88.7983, 38.4766) -> (88.4057, 36.5567) centre (88.798, 37.4766) ccw
  arc A69 (104.0793, 30.6226) -> (104.7095, 30.5207) centre (104.7098, 32.5207) ccw
  arc A70 (109.7552, 38.3866) -> (109.3532, 38.4711) centre (109.353, 37.4711) ccw
  arc A71 (127.5526, 30.5176) -> (127.7097, 31.4923) centre (127.5527, 31.0176) ccw
  line L80 (104.7095, 30.5207) -> (127.5526, 30.5176)
  line L81 (109.7552, 38.3866) -> (127.7097, 31.4923)
  line L82 (104.0793, 30.6226) -> (88.4057, 36.5567)
  line L83 (88.7983, 38.4766) -> (109.3532, 38.4711)
  arc A72 (171.4264, 28.1274) -> (170.2297, 28.0978) centre (170.8752, 26.2048) ccw
  arc A73 (170.2313, 22.9205) -> (171.4285, 22.8907) centre (170.8773, 24.8133) ccw
  arc A74 (164.315, 25.9784) -> (164.3149, 25.0423) centre (164.491, 25.5103) ccw
  arc A75 (180.7426, 25.0159) -> (180.7426, 26.0016) centre (180.6583, 25.5088) ccw
  line L84 (171.4264, 28.1274) -> (180.7426, 26.0016)
  line L85 (180.7426, 25.0159) -> (171.4285, 22.8907)
  line L86 (170.2313, 22.9205) -> (164.3149, 25.0423)
  line L87 (164.315, 25.9784) -> (170.2297, 28.0978)
  arc A76 (143.064, 22.9245) -> (144.2612, 22.8947) centre (143.71, 24.8173) ccw
  arc A77 (144.2591, 28.1314) -> (143.0624, 28.1018) centre (143.7079, 26.2088) ccw
  arc A78 (153.5753, 25.0199) -> (153.5753, 26.0056) centre (153.491, 25.5127) ccw
  arc A79 (137.1477, 25.9823) -> (137.1476, 25.0463) centre (137.3236, 25.5143) ccw
  line L88 (144.2591, 28.1314) -> (153.5753, 26.0056)
  line L89 (153.5753, 25.0199) -> (144.2612, 22.8947)
  line L90 (143.064, 22.9245) -> (137.1476, 25.0463)
  line L91 (137.1477, 25.9823) -> (143.0624, 28.1018)
  arc A80 (115.8967, 22.9284) -> (117.0938, 22.8987) centre (116.5427, 24.8212) ccw
  arc A81 (117.0917, 28.1353) -> (115.8951, 28.1058) centre (116.5406, 26.2128) ccw
  arc A82 (109.9804, 25.9863) -> (109.9803, 25.0503) centre (110.1563, 25.5183) ccw
  arc A83 (126.408, 25.0239) -> (126.408, 26.0095) centre (126.3236, 25.5167) ccw
  line L92 (117.0917, 28.1353) -> (126.408, 26.0095)
  line L93 (117.0938, 22.8987) -> (126.408, 25.0239)
  line L94 (115.8967, 22.9284) -> (109.9803, 25.0503)
  line L95 (109.9804, 25.9863) -> (115.8951, 28.1058)
  arc A84 (22.9928, 27.1102) -> (22.9928, 23.9508) centre (30.8353, 25.5305) ccw
  arc A85 (160.6807, 30.5132) -> (160.8378, 31.4879) centre (160.6808, 31.0132) ccw
  arc A86 (121.9398, 38.4677) -> (121.5472, 36.5479) centre (121.9395, 37.4677) ccw
  arc A87 (142.8967, 38.3777) -> (142.4947, 38.4622) centre (142.4945, 37.4622) ccw
  arc A88 (137.2074, 30.6182) -> (137.8377, 30.5162) centre (137.838, 32.5162) ccw
  line L96 (142.8967, 38.3777) -> (160.8378, 31.4879)
  line L97 (160.6807, 30.5132) -> (137.8377, 30.5162)
  line L98 (137.2074, 30.6182) -> (121.5472, 36.5479)
  line L99 (121.9398, 38.4677) -> (142.4947, 38.4622)
  arc A89 (55.2612, 14.4889) -> (55.6533, 12.569) centre (55.6533, 13.569) ccw
  arc A90 (94.5799, 19.5472) -> (94.4232, 20.522) centre (94.4231, 20.022) ccw
  arc A91 (71.58, 20.5251) -> (70.95, 20.4233) centre (71.5798, 18.5251) ccw
  arc A92 (76.2083, 12.569) -> (76.6102, 12.6534) centre (76.2083, 13.569) ccw
  line L100 (76.6102, 12.6534) -> (94.5799, 19.5472)
  line L101 (94.4232, 20.522) -> (71.58, 20.5251)
  line L102 (70.95, 20.4233) -> (55.2612, 14.4889)
  line L103 (55.6533, 12.569) -> (76.2083, 12.569)
  arc A93 (88.4027, 14.4889) -> (88.7948, 12.569) centre (88.7948, 13.569) ccw
  arc A94 (127.7081, 19.5428) -> (127.5513, 20.5176) centre (127.5512, 20.0176) ccw
  arc A95 (104.7082, 20.5207) -> (104.078, 20.4189) centre (104.7079, 18.5207) ccw
  arc A96 (109.3498, 12.569) -> (109.7517, 12.6534) centre (109.3498, 13.569) ccw
  line L104 (109.7517, 12.6534) -> (127.7081, 19.5428)
  line L105 (127.5513, 20.5176) -> (104.7082, 20.5207)
  line L106 (104.078, 20.4189) -> (88.4027, 14.4889)
  line L107 (88.7948, 12.569) -> (109.3498, 12.569)
  arc A97 (121.5442, 14.4889) -> (121.9363, 12.569) centre (121.9363, 13.569) ccw
  arc A98 (160.8362, 19.5384) -> (160.6794, 20.5132) centre (160.6793, 20.0132) ccw
  arc A99 (137.8364, 20.5162) -> (137.206, 20.4144) centre (137.8361, 18.5162) ccw
  arc A100 (142.4913, 12.569) -> (142.8932, 12.6534) centre (142.4913, 13.569) ccw
  line L108 (142.8932, 12.6534) -> (160.8362, 19.5384)
  line L109 (160.6794, 20.5132) -> (137.8364, 20.5162)
  line L110 (137.206, 20.4144) -> (121.5442, 14.4889)
  line L111 (121.9363, 12.569) -> (142.4913, 12.569)
  arc A101 (190.2846, 21.2083) -> (188.105, 23.2002) centre (188.2846, 21.2083) ccw
  arc A102 (188.3846, 14.6417) -> (190.2846, 16.5417) centre (188.3846, 16.5417) ccw
  arc A103 (160.1468, 15.6085) -> (160.3303, 14.6434) centre (160.3303, 15.1434) ccw
  line L112 (190.2846, 16.5417) -> (190.2846, 21.2083)
  line L113 (188.3846, 14.6417) -> (160.3303, 14.6434)
  arc A104 (188.105, 23.2002) -> (160.1468, 15.6085) centre (195.5628, -59.5415) ccw
  arc A105 (190.2846, 34.4758) -> (188.3846, 36.3758) centre (188.3846, 34.4758) ccw
  arc A106 (188.105, 27.8173) -> (190.2846, 29.8092) centre (188.2846, 29.8092) ccw
  arc A107 (160.3303, 36.3741) -> (160.1468, 35.409) centre (160.3303, 35.8741) ccw
  line L114 (160.3303, 36.3741) -> (188.3846, 36.3758)
  line L115 (190.2846, 34.4758) -> (190.2846, 29.8092)
  arc A108 (160.1468, 35.409) -> (188.105, 27.8173) centre (195.5628, 110.559) ccw
  arc A109 (5.9875, 8.5088) -> (41.2735, 0) centre (43.8737, 88.2038) ccw
  arc A110 (41.2735, 51.0175) -> (5.9833, 42.5088) centre (43.8792, -37.2276) ccw
  arc A111 (88.7294, 22.9284) -> (89.9265, 22.8987) centre (89.3754, 24.8212) ccw
  arc A112 (89.9244, 28.1353) -> (88.7277, 28.1058) centre (89.3732, 26.2128) ccw
  arc A113 (82.8131, 25.9863) -> (82.8129, 25.0503) centre (82.989, 25.5183) ccw
  arc A114 (99.2406, 25.0239) -> (99.2406, 26.0095) centre (99.1563, 25.5167) ccw
  line L116 (89.9244, 28.1353) -> (99.2406, 26.0095)
  line L117 (89.9265, 22.8987) -> (99.2406, 25.0239)
  line L118 (88.7294, 22.9284) -> (82.8129, 25.0503)
  line L119 (82.8131, 25.9863) -> (88.7277, 28.1058)
  line L120 (197.1246, 28.9288) -> (197.1246, 34.4758)
  line L121 (210.561, 34.4758) -> (210.561, 28.9288)
  arc A115 (197.1246, 22.0888) -> (197.1246, 28.9288) centre (193.6586, 25.5088) ccw
  arc A116 (199.0246, 36.3758) -> (197.1246, 34.4758) centre (199.0246, 34.4758) ccw
  arc A117 (210.561, 34.4758) -> (208.661, 36.3758) centre (208.661, 34.4758) ccw
  line L122 (208.661, 36.3758) -> (199.0246, 36.3758)
  arc A118 (197.1246, 22.0888) -> (197.1246, 28.9288) centre (193.6586, 25.5088) ccw
  arc A119 (210.561, 28.9288) -> (210.561, 22.0888) centre (213.981, 25.5088) ccw
  line L123 (210.561, 22.0888) -> (210.561, 16.5417)
  line L124 (208.661, 14.6417) -> (199.0246, 14.6417)
  line L125 (197.1246, 16.5417) -> (197.1246, 22.0888)
  arc A120 (197.1246, 16.5417) -> (199.0246, 14.6417) centre (199.0246, 16.5417) ccw
  arc A121 (208.661, 14.6417) -> (210.561, 16.5417) centre (208.661, 16.5417) ccw
  arc A122 (217.401, 22.0888) -> (217.401, 28.9288) centre (213.981, 25.5088) ccw
  arc A123 (230.321, 28.9288) -> (230.321, 22.0888) centre (233.741, 25.5088) ccw
  arc A124 (229.3266, 18.804) -> (230.321, 20.4743) centre (228.421, 20.4743) ccw
  arc A125 (217.401, 16.5417) -> (219.2195, 14.6434) centre (219.301, 16.5417) ccw
  arc A126 (221.249, 14.6434) -> (222.0731, 14.8714) centre (221.1675, 16.5417) ccw
  arc A127 (217.401, 22.0888) -> (217.401, 28.9288) centre (213.981, 25.5088) ccw
  arc A128 (219.301, 36.3758) -> (217.401, 34.4758) centre (219.301, 34.4758) ccw
  arc A129 (222.0731, 36.1461) -> (221.1675, 36.3758) centre (221.1675, 34.4758) ccw
  line L126 (217.401, 28.9288) -> (217.401, 34.4758)
  line L127 (219.301, 36.3758) -> (221.1675, 36.3758)
  line L128 (222.0731, 36.1461) -> (229.3266, 32.2135)
  line L129 (230.321, 30.5432) -> (230.321, 28.9288)
  line L130 (230.321, 22.0888) -> (230.321, 20.4743)
  line L131 (229.3266, 18.804) -> (222.0731, 14.8714)
  line L132 (221.249, 14.6434) -> (219.2195, 14.6434)
  line L133 (217.401, 16.5417) -> (217.401, 22.0888)
  line L134 (49.8854, 35.7167) -> (71.4567, 27.9227)
  arc A130 (71.4561, 23.1317) -> (71.4567, 27.9227) centre (70.7412, 25.5273) ccw
  line L135 (71.4561, 23.1317) -> (49.8854, 15.3443)
  arc A131 (45.5743, 16.2309) -> (49.8854, 15.3443) centre (48.4027, 19.0594) ccw
  line L136 (45.5743, 16.2309) -> (39.6636, 22.1416)
  arc A132 (39.1172, 23.9508) -> (39.6636, 22.1416) centre (41.0778, 23.5558) ccw
  arc A133 (39.1172, 23.9508) -> (39.1172, 27.1102) centre (31.2747, 25.5305) ccw
  arc A134 (39.6636, 28.9194) -> (39.1172, 27.1102) centre (41.0778, 27.5052) ccw
  arc A135 (49.8854, 35.7167) -> (45.5743, 34.8301) centre (48.4027, 32.0016) ccw
  line L137 (39.6636, 28.9194) -> (45.5743, 34.8301)
  line L138 (6.7874, 36.5088) -> (12.7618, 36.5088)
  arc A136 (16.2903, 35.0513) -> (12.7618, 36.5088) centre (12.7618, 31.5088) ccw
  line L139 (16.2903, 35.0513) -> (22.4464, 28.9194)
  arc A137 (22.9928, 27.1102) -> (22.4464, 28.9194) centre (21.0322, 27.5052) ccw
  arc A138 (22.9928, 27.1102) -> (22.9928, 23.9508) centre (30.8353, 25.5305) ccw
  arc A139 (22.4464, 22.1416) -> (22.9928, 23.9508) centre (21.0322, 23.5558) ccw
  line L140 (22.4464, 22.1416) -> (16.278, 15.9732)
  arc A140 (12.7425, 14.5088) -> (16.278, 15.9732) centre (12.7425, 19.5088) ccw
  arc A141 (4.9392, 15.7445) -> (6.7874, 14.5088) centre (6.7874, 16.5088) ccw
  line L141 (12.7425, 14.5088) -> (6.7874, 14.5088)
  arc A142 (4.9392, 35.273) -> (4.9392, 15.7445) centre (28.5524, 25.5088) ccw
  arc A143 (6.7874, 36.5088) -> (4.9392, 35.273) centre (6.7874, 34.5088) ccw
  arc A144 (29.4753, 17.4683) -> (27.6661, 16.9219) centre (29.0804, 15.5077) ccw
  arc A145 (29.4753, 17.4683) -> (32.6348, 17.4683) centre (31.055, 25.3108) ccw
  arc A146 (34.4439, 16.9219) -> (32.6348, 17.4683) centre (33.0297, 15.5077) ccw
  line L142 (34.4439, 16.9219) -> (38.1065, 13.2594)
  arc A147 (37.3994, 11.5523) -> (38.1065, 13.2594) centre (37.3994, 12.5523) ccw
  line L143 (37.3994, 11.5523) -> (24.7107, 11.5523)
  arc A148 (24.0036, 13.2594) -> (24.7107, 11.5523) centre (24.7107, 12.5523) ccw
  line L144 (24.0036, 13.2594) -> (27.6661, 16.9219)
  line L145 (16.9395, 6.8135) -> (40.3396, 2.2987)
  point P0 (0, 0)
  point P1 (99.1563, 25.5207)
  constraints: 292 end point, 281 point on circle, 149 centre point, 82 tangent, 36 horizontal, 25 vertical, 18 collinear, 11 concentric, 5 parallel, 5 perpendicular, 3 coincident, 1 equal length, 342 other
extrude "Extrusion1" add sketch "Sketch1" against normal blind 2
body "Solid1"
